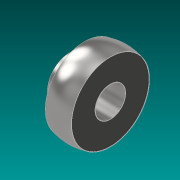
# Autodesk Inventor part: conische lager
Saved by Autodesk Inventor 2020.3 (Build 243373000, 373)
## iProperties
Created: 2020-05-25
Part Number: conische lager
Material: Stainless Steel
Document SubType Name: Modeling
Designer: Svend
Density: 8 g/cm^3
Appearance: Semi-Polished
Author: Svend
Autodesk Inventor part; units mm, degrees
ref_plane "YZ Plane" through (0, 0, 0) normal (1, 0, 0) x (0, 1, 0)
ref_plane "XZ Plane" through (0, 0, 0) normal (0, 1, 0) x (-1, 0, 0)
ref_plane "XY Plane" through (0, 0, 0) normal (0, 0, 1) x (1, 0, 0)
sketch "Sketch2" plane through (0, 0, 0) normal (0, 0, 1) x (1, 0, 0)
  arc A0 (3.5, 10.5) -> (-3.5, 10.5) centre (0, -1.5) ccw
  line L0 (3.5, 10.5) -> (3.5, 4)
  line L1 (3.5, 0) -> (-7.5, 0)
  line L2 (-7.5, 5.9) -> (-3.5, 5.9)
  line L3 (-3.5, 5.9) -> (-3.5, 10.5)
  line L4 (-7.5, 4) -> (3.5, 4)
  line L5 (-7.5, 4) -> (-7.5, 5.9)
  point P0 (0, 0)
  point P1 (0, 11)
  point P2 (-7.5, 4.95)
  dimension "d1" = 11
  dimension "d2" = 3.5
  dimension "d3" = 10.5
  dimension "d4" = 3.5
  dimension "d5" = 5.9
  dimension "d6" = 11
  dimension "d7" = 4
  constraints: 12 end point, 4 vertical alignment, 3 horizontal alignment, 3 perpendicular, 3 point on circle, 2 vertical, 1 centre point, 1 midpoint, 1 point on line
  measures "d1" distance of point (0, 0) point (0, 11)
  measures "d2" horizontal distance of point (0, 11) L0.start
  measures "d3" vertical distance of point (0, 0) L0.start
  measures "d4" horizontal distance of point (0, 11) L3.end
  measures "d5" distance between parallel lines of L1 L2
  measures "d6" distance of L1.start L1.end
  measures "d7" distance between parallel lines of L1 L4
revolve "Revolution1" add sketch "Sketch2" angle 360 about axis through (3.5, 0, 0) along (-1, 0, 0)
sketch "Sketch3" plane through (0, 0, 0) normal (0, 1, 0) x (-1, 0, 0)
  line L0 (7.5, 5.9) -> (7.5, -5.9) projected
  line L1 (3.5, 5.9) -> (3.5, -5.9) projected
  point P0 (0, 0)
  point P1 (5.5, 0)
  dimension "d9" = 2
  constraints: 1 horizontal alignment
  measures "d9" distance from line of point (5.5, 0) L1
hole "Hole1" at (-5.5, 0, 0) direction (0, 1, 0) diameter 2.459 end through all thread size "M3x0.5" class "6H" standard "ISO Metric profile"
pattern_circular "Circular Pattern1" count 2 over 120 about axis through (-2, 0, 0) along (1, 0, 0) of "Hole1"
sketch "Sketch4" plane through (-3.5, 0, 0) normal (-1, 0, 0) x (0, 0, 1)
  circle A0 centre (0, 0) radius 5.9 projected
  circle A1 centre (0, 0) radius 10.5 projected
  circle A2 centre (0, 0) radius 6
  circle A3 centre (0, 0) radius 10.4
  point P0 (0, 0)
  dimension "d20" = 0.1
  dimension "d21" = 0.1
  constraints: 2 centre point
  measures "d20" radial gap between concentric circles of A0 A2
  measures "d21" radial gap between concentric circles of A1 A3
sketch "Sketch4 outline for Extrusion1" plane through (-3.5, 0, 0) normal (-1, 0, 0) x (0, 0, 1)
  circle A0 centre (0, 0) radius 10.4
  circle A1 centre (0, 0) radius 6
extrude "Extrusion1" cut sketch "Sketch4 outline for Extrusion1" against normal blind 0.1
sketch "Sketch5" plane through (3.5, 0, 0) normal (1, 0, 0) x (0, 0, -1)
  circle A0 centre (0, 0) radius 10.5 projected
  circle A1 centre (0, 0) radius 4 projected
  circle A2 centre (0, 0) radius 10.4
  circle A3 centre (0, 0) radius 4.1
  point P0 (0, 0)
  dimension "d24" = 0.1
  dimension "d25" = 0.1
  constraints: 2 centre point
  measures "d24" radial gap between concentric circles of A0 A2
  measures "d25" radial gap between concentric circles of A1 A3
sketch "Sketch5 outline for Extrusion2" plane through (3.5, 0, 0) normal (1, 0, 0) x (0, 0, -1)
  circle A0 centre (0, 0) radius 10.4
  circle A1 centre (0, 0) radius 4.1
extrude "Extrusion2" cut sketch "Sketch5 outline for Extrusion2" against normal blind 0.1
equation "\"d4\" = d2"
body "Solid1"
